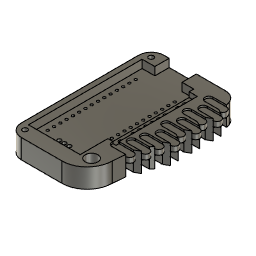
2020_10_03_Arduino Nano Paint Capacitive v6 (Autodesk Fusion 360 design; units mm, degrees)
Autodesk Fusion 360 part; units mm, degrees
(part 1 of 2)
sketch "Measure_ArduinoNano" plane through (0, 0, 0) normal (0, 0, 1) x (1, 0, 0)
  line L0 (-13.9477, 37.28) -> (-13.7477, 37.48)
  line L1 (-4.7943, 37.48) -> (-4.5943, 37.28)
  line L2 (-4.7943, 42.88) -> (-4.5943, 42.68)
  line L3 (-13.9477, 42.68) -> (-13.7477, 42.88)
  line L4 (-18.542, 43.18) -> (-18.542, 0)
  line L5 (-6.771, 0) -> (0, 0)
  line L6 (-17.018, 12.156) -> (-17.018, 11.156)
  line L7 (-12.271, 41.88) -> (-13.7477, 41.88)
  line L8 (-6.771, 18.0694) -> (-6.771, 13.9686)
  line L9 (-6.271, 42.88) -> (-4.7943, 42.88)
  arc A0 (-13.9477, 42.08) -> (-13.9477, 42.68) centre (-14.2477, 42.38) ccw
  arc A1 (-4.5943, 37.28) -> (-4.5943, 36.68) centre (-4.2943, 36.98) ccw
  circle A2 centre (-1.524, 9.156) radius 0.5
  line L10 (-13.7477, 41.88) -> (-13.9477, 42.08)
  line L11 (-12.5236, 31.2001) -> (-12.133, 30.8096)
  line L12 (-12.271, 36.18) -> (-12.271, 36.48)
  line L13 (-4.5943, 42.08) -> (-4.7943, 41.88)
  circle A3 centre (-17.018, 4.156) radius 0.5
  line L14 (-18.542, 0) -> (-11.771, 0)
  arc A4 (-13.9477, 36.68) -> (-13.9477, 37.28) centre (-14.2477, 36.98) ccw
  line L15 (0, 43.18) -> (-6.271, 43.18)
  arc A5 (-4.7943, 36.48) -> (-6.271, 36.48) centre (-5.5326, 35.7416) ccw
  line L16 (-6.271, 43.18) -> (-6.271, 42.88)
  arc A6 (-13.7477, 37.48) -> (-12.271, 37.48) centre (-13.0093, 38.2183) ccw
  line L17 (-6.271, 36.48) -> (-6.271, 36.18)
  line L18 (-13.7477, 36.48) -> (-13.9477, 36.68)
  arc A7 (-12.2912, 24.6445) -> (-12.2912, 24.9274) centre (-12.1497, 24.7859) cw
  line L19 (-4.5943, 36.68) -> (-4.7943, 36.48)
  arc A8 (-4.5943, 42.68) -> (-4.5943, 42.08) centre (-4.2943, 42.38) ccw
  line L20 (-6.271, 41.88) -> (-6.271, 37.48)
  arc A9 (-4.7943, 41.88) -> (-6.271, 41.88) centre (-5.5326, 41.1416) ccw
  line L21 (-6.271, 36.18) -> (-12.271, 36.18)
  line L22 (-12.271, 36.48) -> (-13.7477, 36.48)
  line L23 (-11.771, 0) -> (-6.771, 0)
  line L24 (-6.271, 37.48) -> (-4.7943, 37.48)
  line L25 (-12.271, 37.48) -> (-12.271, 41.88)
  line L26 (0, 0) -> (0, 43.18)
  line L27 (-1.524, 21.656) -> (-1.024, 21.656)
  line L28 (-6.771, 13.9686) -> (-11.771, 13.9686)
  line L29 (-7.771, 0.9965) -> (-6.511, 0.9965)
  circle A10 centre (-17.018, 9.156) radius 0.5
  circle A11 centre (-1.524, 24.156) radius 0.5
  arc A12 (-12.0012, 24.6374) -> (-12.2841, 24.6374) centre (-12.1427, 24.7789) cw
  circle A13 centre (-1.524, 6.656) radius 0.889
  line L30 (0, 43.18) -> (-18.542, 43.18)
  circle A14 centre (-1.524, 11.656) radius 0.5
  line L31 (-12.271, 42.88) -> (-12.271, 43.18)
  circle A15 centre (-17.018, 19.156) radius 0.5
  line L32 (-11.771, 13.9686) -> (-11.771, 18.0694)
  circle A16 centre (-1.524, 14.156) radius 0.5
  line L33 (-16.518, 19.156) -> (-17.018, 19.156)
  circle A17 centre (-7.271, 3.0017) radius 0.76
  arc A18 (-12.8135, 30.9102) -> (-12.8135, 31.1931) centre (-12.6721, 31.0517) cw
  circle A19 centre (-1.524, 24.156) radius 0.889
  line L34 (-12.271, 43.18) -> (-18.542, 43.18)
  line L35 (-11.771, 18.0694) -> (-6.771, 18.0694)
  line L36 (-6.3515, 30.7521) -> (-5.9609, 31.1427)
  line L37 (-12.133, 30.8096) -> (-12.4229, 30.5196)
  line L38 (-12.4635, 4.2) -> (-6.0786, 4.2)
  circle A20 centre (-17.018, 6.656) radius 0.5
  arc A21 (-5.671, 31.1356) -> (-5.671, 30.8528) centre (-5.8124, 30.9942) cw
  line L39 (-5.6781, 31.1427) -> (-5.671, 31.1356)
  circle A22 centre (-17.018, 14.156) radius 0.889
  circle A23 centre (-17.018, 6.656) radius 0.889
  line L40 (-1.524, 19.156) -> (-1.024, 19.156)
  arc A24 (-13.7477, 42.88) -> (-12.271, 42.88) centre (-13.0093, 43.6183) ccw
  line L41 (-18.542, 43.18) -> (0, 43.18)
  line L42 (-11.9006, 25.3179) -> (-11.6107, 25.028)
  line L43 (-5.671, 30.8528) -> (-6.0616, 30.4622)
  line L44 (-1.524, 24.156) -> (-1.024, 24.156)
  line L45 (-12.2841, 24.6374) -> (-12.2912, 24.6445)
  circle A25 centre (-17.018, 14.156) radius 0.5
  line L46 (-15.829, 4.2) -> (-2.8014, 4.2)
  circle A26 centre (-17.018, 31.656) radius 0.889
  line L47 (-6.0616, 30.4622) -> (-6.3515, 30.7521)
  circle A27 centre (-17.018, 9.156) radius 0.889
  circle A28 centre (-17.018, 16.656) radius 0.889
  line L48 (-12.2912, 24.9274) -> (-11.9006, 25.3179)
  arc A29 (-5.9609, 31.1427) -> (-5.6781, 31.1427) centre (-5.8195, 31.0013) cw
  circle A30 centre (-1.524, 16.656) radius 0.5
  line L49 (-7.271, 0.2361) -> (-7.271, 1.7561)
  line L50 (-6.0786, 4.2) -> (-6.0786, 0)
  circle A31 centre (-9.271, 3) radius 0.76
  arc A32 (-12.8065, 31.2001) -> (-12.5236, 31.2001) centre (-12.665, 31.0587) cw
  circle A33 centre (-1.524, 16.656) radius 0.889
  circle A34 centre (-1.524, 19.156) radius 0.5
  circle A35 centre (-17.018, 34.156) radius 0.889
  circle A36 centre (-17.018, 11.656) radius 0.5
  line L51 (-9.1417, 23.3921) -> (-9.4003, 23.3921)
  line L52 (-12.4635, 0) -> (-12.4635, 4.2)
  line L53 (-6.0786, 0) -> (-12.4635, 0)
  line L54 (-12.7703, 26.1877) -> (-13.1609, 25.7971)
  line L55 (-11.6107, 25.028) -> (-12.0012, 24.6374)
  circle A37 centre (-17.018, 11.656) radius 0.889
  circle A38 centre (-1.524, 9.156) radius 0.889
  line L56 (-12.8135, 31.1931) -> (-12.8065, 31.2001)
  line L57 (-12.4229, 30.5196) -> (-12.8135, 30.9102)
  circle A39 centre (-1.524, 14.156) radius 0.889
  arc A40 (-9.5417, 32.9093) -> (-9.4003, 32.9678) centre (-9.4003, 32.7678) cw
  line L58 (-8.0618, 33.5265) -> (-7.9903, 33.4549)
  arc A41 (-8.3447, 33.5265) -> (-8.0618, 33.5265) centre (-8.2033, 33.385) cw
  arc A42 (-6.8307, 32.2953) -> (-6.8307, 32.0124) centre (-6.9721, 32.1539) cw
  circle A43 centre (-17.018, 19.156) radius 0.889
  arc A44 (-4.5417, 28.4507) -> (-4.4831, 28.3093) centre (-4.6831, 28.3093) cw
  circle A45 centre (-1.524, 36.656) radius 0.889
  line L59 (-6.9313, 31.3319) -> (-6.5407, 31.7225)
  line L60 (-7.2212, 31.6218) -> (-7.5112, 31.9118)
  line L61 (-6.2508, 31.4326) -> (-6.6414, 31.042)
  arc A46 (-7.4679, 23.7102) -> (-7.4679, 23.4274) centre (-7.6094, 23.5688) cw
  line L62 (-4.4831, 28.3093) -> (-4.4831, 28.0507)
  line L63 (-17.518, 6.656) -> (-16.518, 6.656)
  arc A47 (-14.0589, 28.3093) -> (-14.0003, 28.4507) centre (-13.8589, 28.3093) cw
  circle A48 centre (-1.524, 39.156) radius 0.889
  line L64 (-13.4508, 26.087) -> (-13.0602, 26.4776)
  line L65 (-7.9903, 33.1721) -> (-8.3809, 32.7815)
  circle A49 centre (-1.524, 31.656) radius 0.5
  arc A50 (-13.1609, 25.7971) -> (-13.4437, 25.7971) centre (-13.3023, 25.9385) cw
  line L66 (-7.5112, 31.9118) -> (-7.1206, 32.3023)
  arc A51 (-9.4003, 23.3921) -> (-9.5417, 23.4507) centre (-9.4003, 23.5921) cw
  arc A52 (-7.1206, 32.3023) -> (-6.8377, 32.3023) centre (-6.9791, 32.1609) cw
  line L67 (-1.524, 36.656) -> (-1.024, 36.656)
  arc A53 (-4.4831, 28.0507) -> (-4.5417, 27.9093) centre (-4.6831, 28.0507) cw
  arc A54 (-7.4105, 32.8751) -> (-7.4105, 32.5923) centre (-7.5519, 32.7337) cw
  line L68 (-9.0003, 32.9093) -> (-4.5417, 28.4507)
  circle A55 centre (-1.524, 4.156) radius 0.889
  line L69 (-6.6414, 31.042) -> (-6.9313, 31.3319)
  line L70 (-7.4105, 32.5923) -> (-7.8011, 32.2017)
  circle A56 centre (-1.524, 4.156) radius 0.5
  line L71 (-13.0602, 26.4776) -> (-12.7703, 26.1877)
  line L72 (-8.7353, 33.1359) -> (-8.3447, 33.5265)
  line L73 (-17.518, 11.656) -> (-16.518, 11.656)
  circle A57 centre (-1.524, 34.156) radius 0.5
  line L74 (-6.8377, 32.3023) -> (-6.8307, 32.2953)
  line L75 (-6.8307, 32.0124) -> (-7.2212, 31.6218)
  line L76 (-14.0589, 28.0507) -> (-14.0589, 28.3093)
  line L77 (-7.8011, 32.2017) -> (-8.091, 32.4916)
  arc A58 (-7.9903, 33.4549) -> (-7.9903, 33.1721) centre (-8.1317, 33.3135) cw
  line L78 (-9.5417, 23.4507) -> (-14.0003, 27.9093)
  line L79 (-1.524, 34.156) -> (-1.024, 34.156)
  arc A59 (-9.0003, 23.4507) -> (-9.1417, 23.3921) centre (-9.1417, 23.5921) cw
  line L80 (-13.4437, 25.7971) -> (-13.4508, 25.8042)
  circle A60 centre (-1.524, 6.656) radius 0.5
  arc A61 (-14.0003, 27.9093) -> (-14.0589, 28.0507) centre (-13.8589, 28.0507) cw
  circle A62 centre (-1.524, 36.656) radius 0.5
  line L81 (-8.3809, 32.7815) -> (-8.7353, 33.1359)
  line L82 (-6.2579, 31.7225) -> (-6.2508, 31.7154)
  circle A63 centre (-17.018, 16.656) radius 0.5
  line L83 (-8.091, 32.4916) -> (-7.7004, 32.8822)
  arc A64 (-6.2508, 31.7154) -> (-6.2508, 31.4326) centre (-6.3922, 31.574) cw
  line L84 (-4.5417, 27.9093) -> (-9.0003, 23.4507)
  line L85 (-7.4176, 32.8822) -> (-7.4105, 32.8751)
  line L86 (-9.4003, 32.9678) -> (-9.1417, 32.9678)
  arc A65 (-6.5407, 31.7225) -> (-6.2579, 31.7225) centre (-6.3993, 31.5811) cw
  line L87 (-12.0199, 1.0002) -> (-10.4999, 1.0002)
  line L88 (-14.0003, 28.4507) -> (-9.5417, 32.9093)
  circle A66 centre (-7.271, 0.9961) radius 0.76
  arc A67 (-7.7004, 32.8822) -> (-7.4176, 32.8822) centre (-7.559, 32.7408) cw
  circle A68 centre (-11.2599, 1.0002) radius 0.76
  arc A69 (-13.4508, 25.8042) -> (-13.4508, 26.087) centre (-13.3094, 25.9456) cw
  arc A70 (-9.1417, 32.9678) -> (-9.0003, 32.9093) centre (-9.1417, 32.7678) cw
  arc A71 (-5.3811, 30.5629) -> (-5.0982, 30.5629) centre (-5.2397, 30.4214) cw
  line L89 (-8.7353, 23.2241) -> (-8.4384, 23.521)
  arc A72 (-5.1557, 25.7396) -> (-5.4385, 25.7396) centre (-5.2971, 25.8811) cw
  line L90 (-4.2789, 26.8993) -> (-4.6695, 27.2899)
  line L91 (-8.0478, 22.8476) -> (-8.0618, 22.8335)
  line L92 (-5.0982, 30.5629) -> (-5.0912, 30.5558)
  line L93 (-6.9888, 24.9706) -> (-6.6989, 25.2605)
  arc A73 (-5.1486, 26.0296) -> (-5.1486, 25.7467) centre (-5.2901, 25.8881) cw
  line L94 (-1.524, 39.156) -> (-1.024, 39.156)
  line L95 (-6.8881, 24.0072) -> (-6.8952, 24.0002)
  arc A74 (-5.0912, 30.5558) -> (-5.0912, 30.2729) centre (-5.2326, 30.4144) cw
  arc A75 (-8.0618, 22.8335) -> (-8.3447, 22.8335) centre (-8.2033, 22.9749) cw
  line L96 (-5.2493, 26.7101) -> (-4.9594, 27)
  line L97 (-5.7717, 30.1723) -> (-5.3811, 30.5629)
  arc A76 (-4.2214, 29.4032) -> (-3.9386, 29.4032) centre (-4.08, 29.2618) cw
  line L98 (-17.018, 37.156) -> (-17.018, 36.156)
  line L99 (-7.5686, 24.3907) -> (-7.2787, 24.6807)
  line L100 (-8.1484, 23.8109) -> (-7.8585, 24.1008)
  line L101 (-7.8585, 24.1008) -> (-7.4679, 23.7102)
  line L102 (-4.8587, 26.3195) -> (-5.2493, 26.7101)
  arc A77 (-4.5688, 26.6094) -> (-4.5688, 26.3265) centre (-4.7102, 26.468) cw
  circle A78 centre (-11.269, 3) radius 0.76
  arc A79 (-4.5113, 29.976) -> (-4.5113, 29.6931) centre (-4.6528, 29.8345) cw
  line L103 (-6.409, 25.5504) -> (-6.119, 25.8403)
  line L104 (-5.5392, 26.4201) -> (-5.1486, 26.0296)
  arc A80 (-6.3154, 24.58) -> (-6.5982, 24.58) centre (-6.4568, 24.7214) cw
  line L105 (-3.9386, 29.4032) -> (-3.9245, 29.3891)
  line L106 (-5.0912, 30.2729) -> (-5.4818, 29.8824)
  line L107 (-6.0184, 25.1598) -> (-6.409, 25.5504)
  arc A81 (-6.8881, 24.2901) -> (-6.8881, 24.0072) centre (-7.0295, 24.1486) cw
  arc A82 (-4.5759, 26.3195) -> (-4.8587, 26.3195) centre (-4.7173, 26.4609) cw
  arc A83 (-6.3083, 24.8699) -> (-6.3083, 24.5871) centre (-6.4497, 24.7285) cw
  line L108 (-7.178, 24.0002) -> (-7.5686, 24.3907)
  line L109 (-5.1486, 25.7467) -> (-5.1557, 25.7396)
  line L110 (-7.4679, 23.4274) -> (-7.475, 23.4203)
  line L111 (-4.5688, 26.3265) -> (-4.5759, 26.3195)
  arc A84 (-5.7355, 25.1598) -> (-6.0184, 25.1598) centre (-5.8769, 25.3012) cw
  line L112 (-4.612, 29.0126) -> (-4.2214, 29.4032)
  line L113 (-3.9245, 26.9708) -> (-3.996, 26.8993)
  line L114 (-4.3151, 28.7157) -> (-4.612, 29.0126)
  line L115 (-7.7579, 23.4203) -> (-8.1484, 23.8109)
  arc A85 (-8.0478, 23.1304) -> (-8.0478, 22.8476) centre (-8.1892, 22.989) cw
  line L116 (-8.3447, 22.8335) -> (-8.7353, 23.2241)
  line L117 (-6.119, 25.8403) -> (-5.7285, 25.4497)
  arc A86 (-7.475, 23.4203) -> (-7.7579, 23.4203) centre (-7.6164, 23.5618) cw
  line L118 (-8.4384, 23.521) -> (-8.0478, 23.1304)
  arc A87 (-3.9245, 29.3891) -> (-3.9245, 29.1063) centre (-4.0659, 29.2477) cw
  line L119 (-6.5982, 24.58) -> (-6.9888, 24.9706)
  line L120 (-7.2787, 24.6807) -> (-6.8881, 24.2901)
  line L121 (-4.9594, 27) -> (-4.5688, 26.6094)
  line L122 (-3.9245, 29.1063) -> (-4.3151, 28.7157)
  arc A88 (-3.996, 26.8993) -> (-4.2789, 26.8993) centre (-4.1375, 27.0407) cw
  line L123 (-5.8291, 26.1302) -> (-5.5392, 26.4201)
  arc A89 (-6.8952, 24.0002) -> (-7.178, 24.0002) centre (-7.0366, 24.1416) cw
  line L124 (-5.7285, 25.1669) -> (-5.7355, 25.1598)
  line L125 (-5.4818, 29.8824) -> (-5.7717, 30.1723)
  line L126 (-4.3151, 27.6443) -> (-3.9245, 27.2537)
  line L127 (-4.6695, 27.2899) -> (-4.3151, 27.6443)
  arc A90 (-5.7285, 25.4497) -> (-5.7285, 25.1669) centre (-5.8699, 25.3083) cw
  arc A91 (-3.9245, 27.2537) -> (-3.9245, 26.9708) centre (-4.0659, 27.1122) cw
  line L128 (-6.3083, 24.5871) -> (-6.3154, 24.58)
  line L129 (-5.4385, 25.7396) -> (-5.8291, 26.1302)
  line L130 (-13.2927, 29.6499) -> (-13.5826, 29.36)
  line L131 (-14.2269, 28.7157) -> (-14.6175, 29.1063)
  line L132 (-13.93, 27.3473) -> (-14.3206, 26.9568)
  circle A92 centre (-1.524, 26.656) radius 0.889
  line L133 (-13.6401, 27.0574) -> (-13.3501, 26.7675)
  line L134 (-4.9019, 29.3025) -> (-5.1918, 29.5924)
  line L135 (-13.3934, 30.6132) -> (-13.3863, 30.6203)
  line L136 (-12.1905, 25.6079) -> (-12.5811, 25.2173)
  line L137 (-14.2269, 27.6443) -> (-13.93, 27.3473)
  line L138 (-4.5184, 29.983) -> (-4.5113, 29.976)
  line L139 (-12.871, 25.5072) -> (-12.4804, 25.8978)
  line L140 (-4.5113, 29.6931) -> (-4.9019, 29.3025)
  line L141 (-14.6175, 27.2537) -> (-14.2269, 27.6443)
  line L142 (-14.0306, 26.6668) -> (-13.6401, 27.0574)
  line L143 (-14.0236, 26.3769) -> (-14.0306, 26.384)
  line L144 (-1.524, 29.156) -> (-1.024, 29.156)
  line L145 (-11.0741, 32.9326) -> (-11.067, 32.9396)
  arc A93 (-13.3934, 30.3304) -> (-13.3934, 30.6132) centre (-13.2519, 30.4718) cw
  circle A94 centre (-1.524, 26.656) radius 0.5
  arc A95 (-12.5811, 25.2173) -> (-12.8639, 25.2173) centre (-12.7225, 25.3587) cw
  line L146 (-14.6034, 26.9568) -> (-14.6175, 26.9708)
  line L147 (-1.524, 26.656) -> (-1.024, 26.656)
  circle A96 centre (-1.524, 29.156) radius 0.889
  arc A97 (-14.3206, 26.9568) -> (-14.6034, 26.9568) centre (-14.462, 27.0982) cw
  line L148 (-13.9732, 30.0334) -> (-13.9661, 30.0405)
  arc A98 (-12.871, 25.2243) -> (-12.871, 25.5072) centre (-12.7296, 25.3658) cw
  arc A99 (-13.9661, 30.0405) -> (-13.6833, 30.0405) centre (-13.8247, 29.8991) cw
  arc A100 (-13.7407, 26.3769) -> (-14.0236, 26.3769) centre (-13.8822, 26.5183) cw
  line L149 (-13.0028, 29.9398) -> (-13.3934, 30.3304)
  line L150 (-11.2633, 31.6793) -> (-11.6539, 32.0699)
  arc A101 (-11.6539, 32.0699) -> (-11.6539, 32.3527) centre (-11.5125, 32.2113) cw
  line L151 (-11.8431, 31.0995) -> (-12.2337, 31.4901)
  line L152 (-11.9438, 31.78) -> (-11.5532, 31.3894)
  circle A102 centre (-17.018, 24.156) radius 0.5
  line L153 (-13.6833, 30.0405) -> (-13.2927, 29.6499)
  circle A103 centre (-1.524, 29.156) radius 0.5
  arc A104 (-12.2337, 31.4901) -> (-12.2337, 31.7729) centre (-12.0923, 31.6315) cw
  line L154 (-11.364, 32.3598) -> (-10.9734, 31.9692)
  line L155 (-5.1918, 29.5924) -> (-4.8013, 29.983)
  line L156 (-11.5532, 31.3894) -> (-11.8431, 31.0995)
  line L157 (-12.4804, 25.8978) -> (-12.1905, 25.6079)
  arc A105 (-12.2266, 31.78) -> (-11.9438, 31.78) centre (-12.0852, 31.6386) cw
  arc A106 (-14.6175, 26.9708) -> (-14.6175, 27.2537) centre (-14.4761, 27.1122) cw
  line L158 (-14.6175, 29.3891) -> (-14.5459, 29.4607)
  line L159 (-13.1034, 30.6203) -> (-12.7129, 30.2297)
  arc A107 (-14.6175, 29.1063) -> (-14.6175, 29.3891) centre (-14.4761, 29.2477) cw
  arc A108 (-13.3863, 30.6203) -> (-13.1034, 30.6203) centre (-13.2449, 30.4789) cw
  arc A109 (-11.6468, 32.3598) -> (-11.364, 32.3598) centre (-11.5054, 32.2184) cw
  line L160 (-11.6539, 32.3527) -> (-11.6468, 32.3598)
  arc A110 (-14.5459, 29.4607) -> (-14.2631, 29.4607) centre (-14.4045, 29.3192) cw
  circle A111 centre (-17.018, 24.156) radius 0.889
  arc A112 (-14.0306, 26.384) -> (-14.0306, 26.6668) centre (-13.8892, 26.5254) cw
  arc A113 (-4.8013, 29.983) -> (-4.5184, 29.983) centre (-4.6598, 29.8416) cw
  line L161 (-14.2631, 29.4607) -> (-13.8725, 29.0701)
  line L162 (-6.6989, 25.2605) -> (-6.3083, 24.8699)
  line L163 (-13.5826, 29.36) -> (-13.9732, 29.7506)
  arc A114 (-11.0741, 32.6497) -> (-11.0741, 32.9326) centre (-10.9326, 32.7911) cw
  line L164 (-12.7129, 30.2297) -> (-13.0028, 29.9398)
  arc A115 (-13.9732, 29.7506) -> (-13.9732, 30.0334) centre (-13.8318, 29.892) cw
  line L165 (-12.8639, 25.2173) -> (-12.871, 25.2243)
  line L166 (-12.2337, 31.7729) -> (-12.2266, 31.78)
  line L167 (-13.8725, 29.0701) -> (-14.2269, 28.7157)
  line L168 (-10.7841, 32.9396) -> (-10.3935, 32.549)
  circle A116 centre (-1.524, 19.156) radius 0.889
  arc A117 (-10.4942, 33.2295) -> (-10.4942, 33.5124) centre (-10.3528, 33.371) cw
  line L169 (-16.518, 24.156) -> (-17.018, 24.156)
  arc A118 (-10.5517, 22.905) -> (-10.5517, 23.1879) centre (-10.4103, 23.0465) cw
  circle A119 centre (-1.524, 31.656) radius 0.9737
  line L170 (-10.451, 23.8684) -> (-10.8416, 23.4778)
  circle A120 centre (-17.018, 29.156) radius 0.889
  circle A121 centre (-17.018, 21.656) radius 0.5
  circle A122 centre (-9.271, 0.998) radius 0.76
  line L171 (0, 43.18) -> (0, 0)
  circle A123 centre (-17.018, 36.656) radius 0.5
  line L172 (-10.9734, 31.9692) -> (-11.2633, 31.6793)
  line L173 (-10.4942, 33.5124) -> (-10.4801, 33.5265)
  arc A124 (-11.4214, 24.0576) -> (-11.7043, 24.0576) centre (-11.5628, 24.199) cw
  circle A125 centre (-17.018, 39.156) radius 0.889
  line L174 (-15.829, 4.2) -> (-15.829, 43.18)
  circle A126 centre (-1.524, 34.156) radius 0.9737
  line L175 (-10.5517, 23.1879) -> (-10.1611, 23.5785)
  circle A127 centre (-1.524, 11.656) radius 0.889
  arc A128 (-10.4801, 33.5265) -> (-10.1973, 33.5265) centre (-10.3387, 33.385) cw
  arc A129 (-10.1973, 22.8335) -> (-10.4801, 22.8335) centre (-10.3387, 22.9749) cw
  arc A130 (-10.8416, 23.4778) -> (-11.1244, 23.4778) centre (-10.983, 23.6192) cw
  line L176 (-16.518, 26.656) -> (-17.018, 26.656)
  line L177 (-16.518, 21.656) -> (-17.018, 21.656)
  line L178 (-11.1315, 23.7677) -> (-10.7409, 24.1583)
  circle A131 centre (-17.018, 21.656) radius 0.889
  line L179 (-10.1973, 33.5265) -> (-9.8067, 33.1359)
  line L180 (-10.7409, 24.1583) -> (-10.451, 23.8684)
  circle A132 centre (-17.018, 39.156) radius 0.5
  line L181 (-18.542, 0) -> (-18.542, 43.18)
  line L182 (-1.524, 31.656) -> (-1.024, 31.656)
  circle A133 centre (-17.018, 26.656) radius 0.5
  line L183 (-13.3501, 26.7675) -> (-13.7407, 26.3769)
  line L184 (-11.1244, 23.4778) -> (-11.1315, 23.4849)
  line L185 (-11.7043, 24.0576) -> (-11.7113, 24.0647)
  circle A134 centre (-17.018, 34.156) radius 0.5
  arc A135 (-11.1315, 23.4849) -> (-11.1315, 23.7677) centre (-10.9901, 23.6263) cw
  line L186 (-10.3935, 32.549) -> (-10.6835, 32.2591)
  line L187 (-2.8014, 4.2) -> (-2.8014, 43.18)
  circle A136 centre (-1.524, 21.656) radius 0.5
  line L188 (-10.1611, 23.5785) -> (-9.8067, 23.2241)
  circle A137 centre (-17.018, 31.656) radius 0.5
  line L189 (-9.8067, 33.1359) -> (-10.1036, 32.839)
  line L190 (-11.7113, 24.3475) -> (-11.3207, 24.7381)
  line L191 (-10.4801, 22.8335) -> (-10.5517, 22.905)
  circle A138 centre (-1.524, 21.656) radius 0.889
  circle A139 centre (-17.018, 26.656) radius 0.889
  arc A140 (-11.067, 32.9396) -> (-10.7841, 32.9396) centre (-10.9256, 32.7982) cw
  line L192 (-2.024, 11.656) -> (-1.024, 11.656)
  line L193 (-17.518, 36.656) -> (-16.518, 36.656)
  line L194 (-11.3207, 24.7381) -> (-11.0308, 24.4482)
  line L195 (-16.518, 14.156) -> (-17.018, 14.156)
  line L196 (-16.518, 16.656) -> (-17.018, 16.656)
  arc A141 (-11.7113, 24.0647) -> (-11.7113, 24.3475) centre (-11.5699, 24.2061) cw
  line L197 (-11.0308, 24.4482) -> (-11.4214, 24.0576)
  line L198 (-16.518, 29.156) -> (-17.018, 29.156)
  circle A142 centre (-17.018, 29.156) radius 0.5
  line L199 (-9.8067, 23.2241) -> (-10.1973, 22.8335)
  line L200 (-10.6835, 32.2591) -> (-11.0741, 32.6497)
  circle A143 centre (-1.524, 39.156) radius 0.5
  circle A144 centre (-17.018, 4.156) radius 0.889
  circle A145 centre (-17.018, 36.656) radius 0.889
  line L201 (-10.1036, 32.839) -> (-10.4942, 33.2295)
sketch "ResistorsLinks" plane through (0, 0, 0) normal (0, 0, 1) x (1, 0, 0)
  line L0 (-1.524, 39.156) -> (-1.024, 39.156)
  line L1 (-17.018, 39.156) -> (-1.524, 39.156) construction
  line L2 (-1.524, 36.656) -> (-14.524, 36.656) construction
  line L3 (-14.524, 36.656) -> (-14.524, 34.156)
  line L4 (-14.524, 34.156) -> (-1.524, 34.156) construction
  line L5 (-1.524, 31.656) -> (-1.024, 31.656)
  line L6 (-17.018, 31.656) -> (-1.524, 31.656) construction
  line L7 (-1.524, 29.156) -> (-17.018, 29.156) construction
  line L8 (-1.524, 26.656) -> (-1.024, 26.656)
  line L9 (-17.018, 26.656) -> (-1.524, 26.656) construction
  line L10 (-16.518, 24.156) -> (-17.018, 24.156)
  line L11 (-1.524, 24.156) -> (-17.018, 24.156) construction
  line L12 (-2.8014, 4.2) -> (-2.8014, 43.18)
  line L13 (-17.018, 21.656) -> (-1.524, 21.656) construction
  line L14 (-17.018, 19.156) -> (-1.524, 19.156) construction
  line L15 (-1.524, 16.656) -> (-14.524, 16.656) construction
  line L16 (-14.524, 16.656) -> (-14.524, 14.156) construction
  line L17 (-14.524, 14.156) -> (-1.524, 14.156) construction
  circle A0 centre (-17.018, 39.156) radius 0.5
  circle A1 centre (-17.018, 39.156) radius 0.889
  circle A2 centre (-1.524, 39.156) radius 0.5
  circle A3 centre (-1.524, 39.156) radius 0.889
  circle A4 centre (-1.524, 36.656) radius 0.5
  circle A5 centre (-1.524, 36.656) radius 0.889
  circle A6 centre (-1.524, 34.156) radius 0.5
  circle A7 centre (-1.524, 34.156) radius 0.9737
  circle A8 centre (-1.524, 31.656) radius 0.5
  circle A9 centre (-1.524, 31.656) radius 0.9737
  circle A10 centre (-1.524, 29.156) radius 0.5
  circle A11 centre (-1.524, 29.156) radius 0.889
  circle A12 centre (-1.524, 26.656) radius 0.5
  circle A13 centre (-1.524, 26.656) radius 0.889
  circle A14 centre (-1.524, 24.156) radius 0.5
  circle A15 centre (-1.524, 24.156) radius 0.889
  circle A16 centre (-1.524, 21.656) radius 0.5
  circle A17 centre (-1.524, 21.656) radius 0.889
  circle A18 centre (-1.524, 19.156) radius 0.5
  circle A19 centre (-1.524, 19.156) radius 0.889
  circle A20 centre (-1.524, 16.656) radius 0.5
  circle A21 centre (-1.524, 16.656) radius 0.889
  circle A22 centre (-1.524, 14.156) radius 0.5
  circle A23 centre (-1.524, 14.156) radius 0.889
  circle A24 centre (-17.018, 19.156) radius 0.5
  circle A25 centre (-17.018, 19.156) radius 0.889
  circle A26 centre (-17.018, 21.656) radius 0.5
  circle A27 centre (-17.018, 21.656) radius 0.889
  circle A28 centre (-17.018, 24.156) radius 0.5
  circle A29 centre (-17.018, 24.156) radius 0.889
  circle A30 centre (-17.018, 26.656) radius 0.5
  circle A31 centre (-17.018, 26.656) radius 0.889
  circle A32 centre (-17.018, 29.156) radius 0.889
  circle A33 centre (-17.018, 29.156) radius 0.5
  circle A34 centre (-17.018, 31.656) radius 0.5
  circle A35 centre (-17.018, 31.656) radius 0.889
  point P0 (-17.018, 39.156)
  point P1 (-1.524, 39.156)
  point P2 (-1.524, 36.656)
  point P3 (-1.524, 34.156)
  point P4 (-17.018, 31.656)
  point P5 (-1.524, 31.656)
  point P6 (-1.524, 29.156)
  point P7 (-17.018, 29.156)
  point P8 (-17.018, 26.656)
  point P9 (-1.524, 26.656)
  point P10 (-1.524, 24.156)
  point P11 (-17.018, 24.156)
  point P12 (-17.018, 21.656)
  point P13 (-1.524, 21.656)
  point P14 (-17.018, 19.156)
  point P15 (-1.524, 19.156)
  point P16 (-1.524, 16.656)
  point P17 (-1.524, 14.156)
  dimension "d1" = 13
  dimension "d3" = 13
  constraint coincident P0 L1.start
  constraint coincident P1 L0.start
  constraint coincident P2 L2.start
  constraint parallel L0 L2
  constraint perpendicular L0 L3
  constraint coincident P3 L4.end
  constraint perpendicular L3 L4
  constraint coincident P4 L6.start
  constraint coincident P5 L5.start
  constraint coincident P6 L7.start
  constraint coincident P7 L7.end
  constraint coincident P8 L9.start
  constraint coincident P9 L8.start
  constraint coincident P10 L11.start
  constraint coincident P11 L10.end
  constraint coincident P12 L13.start
  constraint coincident P13 L13.end
  constraint coincident P14 L14.start
  constraint coincident P15 L14.end
  constraint coincident P16 L15.start
  constraint perpendicular L12 L15
  constraint perpendicular L15 L16
  constraint coincident P17 L17.end
  constraint perpendicular L12 L17
  constraint concentric A20 A21
  constraint concentric A26 A27
  constraint concentric A28 A29
  constraint concentric A32 A33
  constraint concentric A34 A35
  measures "d1" distance of P2 L2.end
  measures "d3" distance of P16 L15.end
sketch "PaintJoints" plane through (0, 0, 0) normal (0, 0, 1) x (1, 0, 0)
  line L0 (-1.524, 39.156) -> (-1.024, 39.156)
  line L1 (-1.524, 39.156) -> (1.476, 39.156) construction
  line L2 (1.476, 39.156) -> (1.476, 14.156) construction
  line L3 (-1.524, 36.656) -> (1.476, 36.656) construction
  line L4 (-1.524, 31.656) -> (1.476, 31.656) construction
  line L5 (-1.524, 29.156) -> (1.476, 29.156) construction
  line L6 (-1.524, 26.656) -> (1.476, 26.656) construction
  line L7 (-1.524, 24.156) -> (1.476, 24.156) construction
  line L8 (-1.524, 21.656) -> (1.476, 21.656) construction
  line L9 (-1.524, 19.156) -> (1.476, 19.156) construction
  line L10 (-1.524, 16.656) -> (1.476, 16.656) construction
  line L11 (-1.524, 14.156) -> (1.476, 14.156) construction
  line L12 (1.476, 40.045) -> (-17.018, 40.045)
  arc A0 (-17.018, 40.045) -> (-17.018, 38.267) centre (-17.018, 39.156) ccw
  line L13 (-17.018, 38.267) -> (1.476, 38.267)
  arc A1 (1.476, 38.267) -> (1.476, 40.045) centre (1.476, 39.156) ccw
  line L14 (1.476, 39.156) -> (-17.018, 39.156) construction
  line L15 (1.476, 37.545) -> (-14.524, 37.545)
  arc A2 (-14.524, 37.545) -> (-14.524, 35.767) centre (-14.524, 36.656) ccw
  line L16 (-14.524, 35.767) -> (1.476, 35.767)
  arc A3 (1.476, 35.767) -> (1.476, 37.545) centre (1.476, 36.656) ccw
  line L17 (1.476, 36.656) -> (-14.524, 36.656) construction
  line L18 (-1.524, 35.1297) -> (-14.524, 35.1297)
  arc A4 (-14.524, 35.1297) -> (-14.524, 33.1823) centre (-14.524, 34.156) ccw
  line L19 (-14.524, 33.1823) -> (-1.524, 33.1823)
  arc A5 (-1.524, 33.1823) -> (-1.524, 35.1297) centre (-1.524, 34.156) ccw
  line L20 (-1.524, 34.156) -> (-14.524, 34.156) construction
  line L21 (-13.635, 34.156) -> (-13.635, 36.656)
  arc A6 (-13.635, 36.656) -> (-15.413, 36.656) centre (-14.524, 36.656) ccw
  line L22 (-15.413, 36.656) -> (-15.413, 34.156)
  arc A7 (-15.413, 34.156) -> (-13.635, 34.156) centre (-14.524, 34.156) ccw
  line L23 (-14.524, 34.156) -> (-14.524, 36.656) construction
  line L24 (1.476, 32.545) -> (-17.018, 32.545)
  arc A8 (-17.018, 32.545) -> (-17.018, 30.767) centre (-17.018, 31.656) ccw
  line L25 (-17.018, 30.767) -> (1.476, 30.767)
  arc A9 (1.476, 30.767) -> (1.476, 32.545) centre (1.476, 31.656) ccw
  line L26 (1.476, 31.656) -> (-17.018, 31.656) construction
  line L27 (1.476, 30.045) -> (-17.018, 30.045)
  arc A10 (-17.018, 30.045) -> (-17.018, 28.267) centre (-17.018, 29.156) ccw
  line L28 (-17.018, 28.267) -> (1.476, 28.267)
  arc A11 (1.476, 28.267) -> (1.476, 30.045) centre (1.476, 29.156) ccw
  line L29 (1.476, 29.156) -> (-17.018, 29.156) construction
  line L30 (1.476, 27.545) -> (-17.018, 27.545)
  arc A12 (-17.018, 27.545) -> (-17.018, 25.767) centre (-17.018, 26.656) ccw
  line L31 (-17.018, 25.767) -> (1.476, 25.767)
  arc A13 (1.476, 25.767) -> (1.476, 27.545) centre (1.476, 26.656) ccw
  line L32 (1.476, 26.656) -> (-17.018, 26.656) construction
  line L33 (1.476, 25.045) -> (-17.018, 25.045)
  arc A14 (-17.018, 25.045) -> (-17.018, 23.267) centre (-17.018, 24.156) ccw
  line L34 (-17.018, 23.267) -> (1.476, 23.267)
  arc A15 (1.476, 23.267) -> (1.476, 25.045) centre (1.476, 24.156) ccw
  line L35 (1.476, 24.156) -> (-17.018, 24.156) construction
  line L36 (1.476, 22.545) -> (-17.018, 22.545)
  arc A16 (-17.018, 22.545) -> (-17.018, 20.767) centre (-17.018, 21.656) ccw
  line L37 (-17.018, 20.767) -> (1.476, 20.767)
  arc A17 (1.476, 20.767) -> (1.476, 22.545) centre (1.476, 21.656) ccw
  line L38 (1.476, 21.656) -> (-17.018, 21.656) construction
  line L39 (1.476, 20.045) -> (-17.018, 20.045)
  arc A18 (-17.018, 20.045) -> (-17.018, 18.267) centre (-17.018, 19.156) ccw
  line L40 (-17.018, 18.267) -> (1.476, 18.267)
  arc A19 (1.476, 18.267) -> (1.476, 20.045) centre (1.476, 19.156) ccw
  line L41 (1.476, 19.156) -> (-17.018, 19.156) construction
  line L42 (1.476, 15.045) -> (-14.524, 15.045)
  arc A20 (-14.524, 15.045) -> (-14.524, 13.267) centre (-14.524, 14.156) ccw
  line L43 (-14.524, 13.267) -> (1.476, 13.267)
  arc A21 (1.476, 13.267) -> (1.476, 15.045) centre (1.476, 14.156) ccw
  line L44 (1.476, 14.156) -> (-14.524, 14.156) construction
  line L45 (-1.524, 17.545) -> (-14.524, 17.545)
  arc A22 (-14.524, 17.545) -> (-14.524, 15.767) centre (-14.524, 16.656) ccw
  line L46 (-14.524, 15.767) -> (-1.524, 15.767)
  arc A23 (-1.524, 15.767) -> (-1.524, 17.545) centre (-1.524, 16.656) ccw
  line L47 (-1.524, 16.656) -> (-14.524, 16.656) construction
  line L48 (-15.413, 16.656) -> (-15.413, 14.156)
  arc A24 (-15.413, 14.156) -> (-13.635, 14.156) centre (-14.524, 14.156) ccw
  line L49 (-13.635, 14.156) -> (-13.635, 16.656)
  arc A25 (-13.635, 16.656) -> (-15.413, 16.656) centre (-14.524, 16.656) ccw
  line L50 (-14.524, 16.656) -> (-14.524, 14.156) construction
  line L51 (7.548, 42.1183) -> (13.048, 42.1183)
  arc A26 (13.048, 42.1183) -> (13.048, 45.2183) centre (13.048, 43.6683) ccw
  line L52 (13.048, 45.2183) -> (7.548, 45.2183)
  arc A27 (7.548, 45.2183) -> (7.548, 42.1183) centre (7.548, 43.6683) ccw
  line L53 (7.548, 43.6683) -> (13.048, 43.6683) construction
  line L54 (15.048, 40.9683) -> (9.548, 40.9683)
  arc A28 (9.548, 40.9683) -> (9.548, 37.8683) centre (9.548, 39.4183) ccw
  arc A29 (15.048, 37.8683) -> (15.048, 40.9683) centre (15.048, 39.4183) ccw
  line L55 (9.548, 37.8683) -> (15.048, 37.8683)
  line L56 (13.048, 36.7183) -> (7.548, 36.7183)
  arc A30 (7.548, 36.7183) -> (7.548, 33.6183) centre (7.548, 35.1683) ccw
  arc A31 (13.048, 33.6183) -> (13.048, 36.7183) centre (13.048, 35.1683) ccw
  line L57 (7.548, 33.6183) -> (13.048, 33.6183)
  line L58 (15.048, 32.4683) -> (9.548, 32.4683)
  arc A32 (9.548, 32.4683) -> (9.548, 29.3683) centre (9.548, 30.9183) ccw
  arc A33 (15.048, 29.3683) -> (15.048, 32.4683) centre (15.048, 30.9183) ccw
  line L59 (9.548, 29.3683) -> (15.048, 29.3683)
  line L60 (13.048, 28.2183) -> (7.548, 28.2183)
  arc A34 (7.548, 28.2183) -> (7.548, 25.1183) centre (7.548, 26.6683) ccw
  arc A35 (13.048, 25.1183) -> (13.048, 28.2183) centre (13.048, 26.6683) ccw
  line L61 (7.548, 25.1183) -> (13.048, 25.1183)
  line L62 (15.048, 23.9683) -> (9.548, 23.9683)
  arc A36 (9.548, 23.9683) -> (9.548, 20.8683) centre (9.548, 22.4183) ccw
  arc A37 (15.048, 20.8683) -> (15.048, 23.9683) centre (15.048, 22.4183) ccw
  line L63 (9.548, 20.8683) -> (15.048, 20.8683)
  line L64 (13.048, 19.7183) -> (7.548, 19.7183)
  arc A38 (7.548, 19.7183) -> (7.548, 16.6183) centre (7.548, 18.1683) ccw
  arc A39 (13.048, 16.6183) -> (13.048, 19.7183) centre (13.048, 18.1683) ccw
  line L65 (7.548, 16.6183) -> (13.048, 16.6183)
  line L66 (12.048, 15.4683) -> (6.548, 15.4683)
  arc A40 (6.548, 15.4683) -> (6.548, 12.3683) centre (6.548, 13.9183) ccw
  arc A41 (12.048, 12.3683) -> (12.048, 15.4683) centre (12.048, 13.9183) ccw
  line L67 (6.548, 12.3683) -> (12.048, 12.3683)
  line L68 (10.048, 11.2183) -> (4.548, 11.2183)
  arc A42 (4.548, 11.2183) -> (4.548, 8.1183) centre (4.548, 9.6683) ccw
  arc A43 (10.048, 8.1183) -> (10.048, 11.2183) centre (10.048, 9.6683) ccw
  line L69 (4.548, 8.1183) -> (10.048, 8.1183)
  line L70 (1.476, 26.656) -> (6.7423, 26.656) construction
  line L71 (4.548, 9.6683) -> (1.476, 14.156) construction
  line L72 (6.548, 13.9183) -> (1.476, 19.156) construction
  line L73 (7.548, 18.1683) -> (1.476, 21.656) construction
  line L74 (9.548, 22.4183) -> (1.476, 24.156) construction
  line L75 (1.476, 29.156) -> (9.548, 30.9183) construction
  line L76 (1.476, 31.656) -> (7.548, 35.1683) construction
  line L77 (1.476, 36.656) -> (9.548, 39.4183) construction
  line L78 (1.476, 39.156) -> (7.548, 43.6683) construction
  circle A44 centre (7.548, 43.6683) radius 1.55
  circle A45 centre (13.048, 43.6683) radius 1.55
  circle A46 centre (15.048, 39.4183) radius 1.55
  circle A47 centre (9.548, 39.4183) radius 1.55
  circle A48 centre (13.048, 35.1683) radius 1.55
  circle A49 centre (7.548, 35.1683) radius 1.55
  circle A50 centre (15.048, 30.9183) radius 1.55
  circle A51 centre (9.548, 30.9183) radius 1.55
  circle A52 centre (13.048, 26.6683) radius 1.55
  circle A53 centre (7.548, 26.6683) radius 1.55
  circle A54 centre (15.048, 22.4183) radius 1.55
  circle A55 centre (9.548, 22.4183) radius 1.55
  circle A56 centre (13.048, 18.1683) radius 1.55
  circle A57 centre (7.548, 18.1683) radius 1.55
  circle A58 centre (12.048, 13.9183) radius 1.55
  circle A59 centre (6.548, 13.9183) radius 1.55
  circle A60 centre (10.048, 9.6683) radius 1.55
  circle A61 centre (4.548, 9.6683) radius 1.55
  line L79 (1.983, 38.4737) -> (8.055, 42.9861)
  line L80 (1.7512, 35.8518) -> (9.8232, 38.6141)
  line L81 (1.9016, 30.9202) -> (7.9736, 34.4325)
  line L82 (1.6573, 28.3255) -> (9.7293, 30.0879)
  line L83 (1.476, 25.806) -> (6.7423, 25.806)
  line L84 (9.7269, 23.2493) -> (1.6549, 24.9869)
  line L85 (7.9714, 18.9054) -> (1.8994, 22.393)
  line L86 (7.1586, 14.5096) -> (2.0866, 19.7473)
  line L87 (5.2494, 10.1485) -> (2.1774, 14.6361)
  line L88 (3.8466, 9.1882) -> (0.7746, 13.6758)
  line L89 (5.9374, 13.327) -> (0.8654, 18.5647)
  line L90 (7.1246, 17.4312) -> (1.0527, 20.9189)
  line L91 (1.476, 27.506) -> (6.7423, 27.506)
  line L92 (9.3691, 21.5873) -> (1.2971, 23.325)
  line L93 (1.2947, 29.9864) -> (9.3667, 31.7488)
  line L94 (1.0504, 32.3918) -> (7.1224, 35.9041)
  line L95 (1.2008, 37.4602) -> (9.2728, 40.2225)
  line L96 (0.969, 39.8382) -> (7.041, 44.3506)
  point P0 (-1.524, 39.156)
  point P1 (-1.524, 36.656)
  point P2 (-1.524, 31.656)
  point P3 (-1.524, 29.156)
  point P4 (-1.524, 26.656)
  point P5 (-1.524, 24.156)
  point P6 (-1.524, 21.656)
  point P7 (-1.524, 19.156)
  point P8 (-1.524, 16.656)
  point P9 (-1.524, 14.156)
  point P10 (-17.018, 39.156)
  point P11 (-14.524, 36.656)
  point P12 (-1.524, 34.156)
  point P13 (-14.524, 34.156)
  point P14 (-17.018, 31.656)
  point P15 (-17.018, 29.156)
  point P16 (-17.018, 26.656)
  point P17 (-17.018, 24.156)
  point P18 (-17.018, 21.656)
  point P19 (-17.018, 19.156)
  point P20 (-14.524, 14.156)
  point P21 (-14.524, 16.656)
  dimension "d4" = 3
  dimension "d5" = 5.5
  dimension "d6" = 3.1
  dimension "d13" = 0.85
  dimension "d14" = 0.85
  dimension "d15" = 0.85
  dimension "d16" = 0.85
  dimension "d17" = 0.85
  dimension "d18" = 0.85
  dimension "d19" = 0.85
  dimension "d20" = 0.85
  dimension "d21" = 0.85
  constraint coincident P0 L0.start
  constraint parallel L0 L1
  constraint perpendicular L1 L2
  constraint coincident P1 L3.start
  constraint coincident L2 L3.end
  constraint perpendicular L2 L3
  constraint coincident P2 L4.start
  constraint coincident L2 L4.end
  constraint perpendicular L2 L4
  constraint coincident P3 L5.start
  constraint coincident L2 L5.end
  constraint perpendicular L2 L5
  constraint coincident P4 L6.start
  constraint midpoint L2 L6.end
  constraint perpendicular L2 L6
  constraint coincident P5 L7.start
  constraint coincident L2 L7.end
  constraint perpendicular L2 L7
  constraint coincident P6 L8.start
  constraint coincident L2 L8.end
  constraint perpendicular L2 L8
  constraint coincident P7 L9.start
  constraint coincident L2 L9.end
  constraint perpendicular L2 L9
  constraint coincident P8 L10.start
  constraint coincident L2 L10.end
  constraint perpendicular L2 L10
  constraint coincident P9 L11.start
  constraint tangent L12 A0
  constraint tangent A0 L13
  constraint parallel L12 L13
  constraint tangent L13 A1
  constraint tangent L12 A1
  constraint coincident P10 A0.centre
  constraint perpendicular L2 L14
  constraint coincident L1.end L2.start
  constraint tangent L15 A2
  constraint tangent A2 L16
  constraint parallel L15 L16
  constraint tangent L16 A3
  constraint tangent L15 A3
  constraint coincident P11 A2.centre
  constraint perpendicular L2 L17
  constraint coincident L3.end A3.centre
  constraint tangent L18 A4
  constraint tangent A4 L19
  constraint parallel L18 L19
  constraint tangent L19 A5
  constraint tangent L18 A5
  constraint coincident P13 A4.centre
  constraint perpendicular L2 L20
  constraint coincident P12 A5.centre
  constraint tangent L21 A6
  constraint tangent A6 L22
  constraint parallel L21 L22
  constraint tangent L22 A7
  constraint tangent L21 A7
  constraint perpendicular L17 L23
  constraint tangent L24 A8
  constraint tangent A8 L25
  constraint parallel L24 L25
  constraint tangent L25 A9
  constraint tangent L24 A9
  constraint coincident P14 A8.centre
  constraint perpendicular L2 L26
  constraint coincident L4.end A9.centre
  constraint tangent L27 A10
  constraint tangent A10 L28
  constraint parallel L27 L28
  constraint tangent L28 A11
  constraint tangent L27 A11
  constraint coincident P15 A10.centre
  constraint perpendicular L2 L29
  constraint coincident L5.end A11.centre
  constraint tangent L30 A12
  constraint tangent A12 L31
  constraint parallel L30 L31
  constraint tangent L31 A13
  constraint tangent L30 A13
  constraint coincident P16 A12.centre
  constraint perpendicular L2 L32
  constraint coincident L6.end A13.centre
  constraint tangent L33 A14
  constraint tangent A14 L34
  constraint parallel L33 L34
  constraint tangent L34 A15
  constraint tangent L33 A15
  constraint coincident P17 A14.centre
  constraint perpendicular L2 L35
  constraint coincident L7.end A15.centre
  constraint tangent L36 A16
  constraint tangent A16 L37
  constraint parallel L36 L37
  constraint tangent L37 A17
  constraint tangent L36 A17
  constraint coincident P18 A16.centre
  constraint perpendicular L2 L38
  constraint coincident L8.end A17.centre
  constraint tangent L39 A18
  constraint tangent A18 L40
  constraint parallel L39 L40
  constraint tangent L40 A19
  constraint tangent L39 A19
  constraint coincident P19 A18.centre
  constraint perpendicular L2 L41
  constraint coincident L9.end A19.centre
  constraint tangent L42 A20
  constraint tangent A20 L43
  constraint parallel L42 L43
  constraint tangent L43 A21
  constraint tangent L42 A21
  constraint coincident P20 A20.centre
  constraint perpendicular L2 L44
  constraint coincident L2.end L11.end
  constraint tangent L45 A22
  constraint tangent A22 L46
  constraint parallel L45 L46
  constraint tangent L46 A23
  constraint tangent L45 A23
  constraint coincident P21 A22.centre
  constraint parallel L10 L47
  constraint tangent L48 A24
  constraint tangent A24 L49
  constraint parallel L48 L49
  constraint tangent L49 A25
  constraint tangent L48 A25
  constraint perpendicular L44 L50
  constraint tangent L51 A26
  constraint tangent A26 L52
  constraint parallel L51 L52
  constraint tangent L52 A27
  constraint tangent L51 A27
  constraint horizontal L53
  constraint parallel L6 L70
  constraint coincident A42.centre L71.start
  constraint coincident A40.centre L72.start
  constraint coincident A38.centre L73.start
  constraint coincident A36.centre L74.start
  constraint coincident A32.centre L75.end
  constraint coincident A30.centre L76.end
  constraint coincident A28.centre L77.end
  constraint coincident A27.centre L53.start
  constraint coincident L52.end A44
  constraint concentric A26 A45
  constraint coincident A26.end A45
  measures "d4" distance of P0 L1.end
  measures "d5" distance of A27.centre A26.centre
  measures "d6" diameter of A26
sketch "Border" plane through (0, 0, 0) normal (0, 0, 1) x (1, 0, 0)
  line L0 (7.9458, 49.881) -> (-16.6051, 49.881)
  line L1 (-21.6051, 44.881) -> (-21.6051, -1.7992)
  line L2 (-16.6051, -6.7992) -> (-0.4432, -6.7992)
  line L3 (12.9458, 12.6427) -> (12.9458, 44.881) construction
  arc A0 (-16.6051, 49.881) -> (-21.6051, 44.881) centre (-16.6051, 44.881) ccw
  arc A1 (12.5923, 46.7277) -> (7.9458, 49.881) centre (7.9458, 44.881) ccw
  arc A2 (7.9458, -6.7992) -> (9.5568, -6.5325) centre (7.9458, -1.7992) ccw
  arc A3 (-21.6051, -1.7992) -> (-16.6051, -6.7992) centre (-16.6051, -1.7992) ccw
  arc A4 (13.048, 42.1183) -> (13.048, 45.2183) centre (13.048, 43.6683) ccw
  circle A5 centre (15.048, 39.4183) radius 1.55
  circle A6 centre (13.048, 35.1683) radius 1.55
  arc A7 (15.048, 29.3683) -> (15.048, 32.4683) centre (15.048, 30.9183) ccw
  arc A8 (13.048, 25.1183) -> (13.048, 28.2183) centre (13.048, 26.6683) ccw
  arc A9 (15.048, 20.8683) -> (15.048, 23.9683) centre (15.048, 22.4183) ccw
  circle A10 centre (15.048, 22.4183) radius 1.55
  arc A11 (13.048, 16.6183) -> (13.048, 19.7183) centre (13.048, 18.1683) ccw
  circle A12 centre (12.048, 13.9183) radius 1.55
  line L4 (12.0907, 15.5174) -> (12.0248, 15.4681)
  circle A13 centre (10.048, 9.6683) radius 1.55
  line L5 (13.0767, 12.7588) -> (12.9458, 12.6427)
  arc A14 (15.048, 37.8683) -> (15.048, 40.9683) centre (15.048, 39.4183) ccw
  circle A15 centre (13.048, 18.1683) radius 1.55
  arc A16 (12.048, 12.3683) -> (12.048, 15.4683) centre (12.048, 13.9183) ccw
  arc A17 (-0.4432, -6.7992) -> (9.5568, 3.2008) centre (-0.4432, 3.2008) ccw
  line L6 (-16.6051, 44.881) -> (-20.1407, 48.4166) construction
  line L7 (-16.6051, -1.7992) -> (-20.4628, -4.9801) construction
  circle A18 centre (-18.3729, 46.6488) radius 1
  circle A19 centre (-18.534, -3.3897) radius 1
  line L8 (12.9458, 44.881) -> (12.5923, 46.7277) construction
  arc A20 (13.048, 42.1183) -> (13.048, 45.2183) centre (13.048, 43.6683) ccw
  arc A21 (15.048, 37.8683) -> (15.048, 40.9683) centre (15.048, 39.4183) ccw
  circle A22 centre (13.048, 35.1683) radius 1.55
  arc A23 (15.048, 29.3683) -> (15.048, 32.4683) centre (15.048, 30.9183) ccw
  arc A24 (13.048, 25.1183) -> (13.048, 28.2183) centre (13.048, 26.6683) ccw
  arc A25 (13.048, 25.1183) -> (13.048, 28.2183) centre (13.048, 26.6683) ccw
  arc A26 (15.048, 20.8683) -> (15.048, 23.9683) centre (15.048, 22.4183) ccw
  circle A27 centre (13.048, 18.1683) radius 1.55
  circle A28 centre (12.048, 13.9183) radius 1.55
  circle A29 centre (10.048, 9.6683) radius 1.55
  arc A30 (13.048, 42.1183) -> (13.048, 45.2183) centre (13.048, 43.6683) ccw
  circle A31 centre (4.5445, 0) radius 2.5
  line L9 (9.9615, 11.2159) -> (12.048, 12.3683)
  line L10 (12.048, 15.4683) -> (13.048, 16.6183)
  line L11 (13.048, 19.7183) -> (15.048, 20.8683)
  line L12 (13.048, 25.1183) -> (15.048, 23.9683)
  line L13 (13.048, 28.2183) -> (15.048, 29.3683)
  line L14 (13.048, 33.6183) -> (15.048, 32.4683)
  line L15 (13.048, 36.7183) -> (15.048, 37.8683)
  line L16 (13.048, 42.1183) -> (15.048, 40.9683)
  arc A32 (12.6247, 46.5581) -> (12.5923, 46.7277) centre (12.1654, 46.5581) ccw
  line L17 (13.048, 45.2183) -> (12.5923, 46.7277)
  line L18 (10.048, 8.1183) -> (9.5568, 3.2008)
  dimension "d35" = 5
  dimension "d36" = 10
  dimension "d37" = 2
  dimension "d38" = 2
  dimension "d45" = 5
  constraint horizontal L0
  constraint vertical L1
  constraint horizontal L2
  constraint vertical L3
  constraint tangent L1 A0
  constraint tangent L0 A0
  constraint tangent L0 A1
  constraint tangent L3 A1
  constraint equal A0 A1
  constraint tangent L3 A2
  constraint tangent L2 A2
  constraint equal A0 A2
  constraint tangent L2 A3
  constraint tangent L1 A3
  constraint equal A0 A3
  constraint coincident A12 L4.end
  constraint coincident A12 L5.start
  constraint tangent L4 A15
  constraint tangent L5 A16
  constraint coincident L2 A2.start
  constraint tangent L2 A17
  constraint coincident A0.centre L6.start
  constraint midpoint A0 L6.end
  constraint coincident A3.centre L7.start
  constraint coincident A3 L7.end
  constraint midpoint L6 A18.centre
  constraint midpoint L7 A19.centre
  constraint coincident A13 L9.start
  constraint coincident A16.start L9.end
  constraint coincident A16.end L10.start
  constraint coincident A11.start L10.end
  constraint coincident A11.end L11.start
  constraint coincident A9.start A26.start
  constraint coincident A9.end A26.end
  constraint parallel L11 L13
  constraint coincident A22 L14.start
  constraint parallel L12 L14
  constraint coincident A22 L15.start
  constraint coincident A14.start A21.start
  constraint parallel L13 L15
  constraint parallel L14 L16
  constraint coincident L8 A32.start
  constraint tangent A1 A32
  constraint coincident A4.end A20.end
  constraint coincident A13 L18.start
  constraint coincident L10 L4.start
  measures "d35" radius of A0
  measures "d36" radius of A17
  measures "d37" diameter of A18
  measures "d38" diameter of A19
  measures "d45" diameter of A31
extrude "Extrude1" add sketch "Border" along normal blind 7.7 contours L0 L1 L2 A0 A1 A3 A4 A5 A6 A7 A8 A10 A12 L4 A13 A15 A17 A20 A22 A23 A24 A25 A27 A28 A29 A30 L9 L10 L11 L12 L13 L14 L15 L16 L17 L18 | A5 A14 A21 | A6 A22 | A13 A29 | A12 A16 A28 | A11 A15 A27 | A9 A10 A26 makes body 1
extrude "Extrude2" cut sketch "PaintJoints" along normal blind 3 bodies 1
sketch "ArduinoNanoHole" plane through (0, 0, 0) normal (0, 0, 1) x (1, 0, 0)
  line L0 (0, 0) -> (0, 43.18)
  line L1 (-18.542, 0) -> (-11.771, 0)
  line L2 (-11.771, 0) -> (-6.771, 0)
  line L3 (-6.771, 0) -> (0, 0)
  line L4 (-18.542, 43.18) -> (-18.542, 0)
  line L5 (-18.542, 43.18) -> (0, 43.18)
  line L6 (-15.829, 4.2) -> (-2.8014, 4.2)
  line L7 (-2.8014, 4.2) -> (-2.8014, 43.18)
  line L8 (-15.829, 4.2) -> (-15.829, 43.18)
  line L9 (-14.4757, 43.18) -> (-3.661, 43.18)
  line L10 (-3.661, 43.18) -> (-3.661, 35.1297)
  line L11 (-3.661, 35.1297) -> (-14.4757, 35.1297)
  line L12 (-14.4757, 35.1297) -> (-14.4757, 43.18)
  line L13 (-1.524, 35.1297) -> (-13.635, 35.1297)
  line L14 (-14.4757, 43.18) -> (-3.661, 43.18)
  line L15 (-3.661, 43.18) -> (-3.661, 49.881)
  line L16 (-3.661, 49.881) -> (-14.4757, 49.881)
  line L17 (-14.4757, 49.881) -> (-14.4757, 43.18)
  line L18 (7.9458, 49.881) -> (-16.6051, 49.881)
  line L19 (-19.542, 44.18) -> (1, 44.18)
  line L20 (1, -1) -> (1, 44.18)
  line L21 (-6.771, -1) -> (1, -1)
  line L22 (-11.771, -1) -> (-6.771, -1)
  line L23 (-19.542, -1) -> (-11.771, -1)
  line L24 (-19.542, 44.18) -> (-19.542, -1)
  dimension "d60" = 1
  constraint horizontal L9
  constraint vertical L10
  constraint horizontal L11
  constraint vertical L12
  constraint coincident L10.end L13
  constraint coincident L5 L9.start
  constraint horizontal L14
  constraint vertical L15
  constraint horizontal L16
  constraint vertical L17
  constraint coincident L15.end L18
extrude "Extrude3" add sketch "ArduinoNanoHole" along normal blind 15 separate body contours L0 L1 L2 L3 L4 L5 L6 L7 L8 | L0 L1 L2 L3 L4 L5 L15 L17 L19 L20 L21 L22 L23 L24 makes body 2
extrude "Extrude4" add sketch "ArduinoNanoHole" along normal blind 15 separate body contours L5 L7 L10 L13 | L5 L9 L10 L11 L12 L13 L14 | L5 L9 L14 L15 L17 L19 | L5 L6 L7 L8 L11 L12 L13 | L15 L16 L17 L18 L19 makes body 3
move_body "Move1" bodies 2 to x (1, 0, 0) y (0, 1, 0) z (0, 0, 1) at (0, 0, 2)
move_body "Move2" bodies 2 3 to x (1, 0, 0) y (0, 1, 0) z (0, 0, 1) at (0, 0, 4.5)
combine "Combine1" operation cut target body 1 tool bodies 2 3
extrude "Extrude5" cut sketch "Measure_ArduinoNano" along normal blind 7.7 contours L6 A36 L73 | L6 A36 L73 | L6 A36 L73 | L6 A36 L73 | A2 | A3 | L29 L49 A66 | L29 L49 A66 | L49 A66 | A10 | A11 | A14 L192 | A14 L192 | A15 | A16 | A17 | A20 L63 | A20 L63 | A25 | A30 | A31 | A34 | A49 | A56 | A57 | A60 | A62 | A63 | L87 A68 | L87 A68 | L98 A123 L193 | L98 A123 L193 | L98 A123 L193 | L98 A123 L193 | A78 | A94 | A102 | A103 | A121 | A122 | A132 | A133 | A134 | A136 | A137 | A142 | A143 bodies 1
extrude "Extrude6" cut sketch "PaintJoints" along normal blind 5 contours A27 A44 | A26 A45 | A28 A47 | A29 A46 | A30 A49 | A31 A48 | A32 A51 | A33 A50 | A34 A53 | A35 A52 | A36 A55 | A37 A54 | A38 A57 | A39 A56 | A40 A59 | A41 A58 | A42 A61 | A43 A60 bodies 1
extrude "Extrude7" add sketch "PaintJoints" along normal blind 0.7 separate body contours A27 A44 | L51 L52 A44 A45 | A26 A45 | A28 A47 | L54 L55 A46 A47 | A29 A46 | A30 A49 | L56 L57 A48 A49 | A31 A48 | A32 A51 | L58 L59 A50 A51 | A33 A50 | A34 A53 | L60 L61 A52 A53 | A35 A52 | A36 A55 | L62 L63 A54 A55 | A37 A54 | A38 A57 | L64 L65 A56 A57 | A39 A56 | A40 A59 | L66 L67 A58 A59 | A41 A58 | A42 A61 | L68 L69 A60 A61 | A43 A60 makes body 4 at (9.3813, 35.685, 0) makes body 5 at (9.3813, 18.685, 0) makes body 6 at (8.3813, 14.435, 0) makes body 7 at (11.3813, 31.435, 0) makes body 8 at (13.2147, 39.935, 0.7) makes body 9 at (11.3813, 22.935, 0) makes body 10 at (6.3813, 10.185, 0.7) makes body 11 at (9.3813, 27.185, 0) makes body 12 at (11.2147, 43.1516, 0)
move_body "Move3" bodies 12 8 4 7 11 9 5 6 10 to x (1, 0, 0) y (0, 1, 0) z (0, 0, 1) at (0, 0, 7)
combine "Combine2" operation cut target body 1 tool bodies 4 6 7 5 10 11 12 9 8